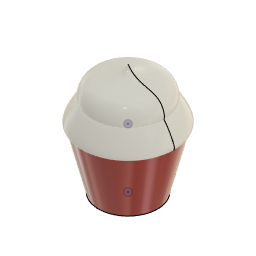
Cupcake v1 (Autodesk Fusion 360 design; units mm, degrees)
Autodesk Fusion 360 part; units mm, degrees
sketch "Sketch1" plane through (0, 0, 0) normal (0, 0, 1) x (1, 0, 0)
ref_plane "WorkPlane2" through (0, 0, 12.7) normal (0, 0, 1) x (1, 0, 0)
sketch "Sketch2" plane through (0, 0, 12.7) normal (0, 0, 1) x (1, 0, 0)
sketch "Sketch3" plane through (0, 0, 0) normal (0, 0, 1) x (1, 0, 0)
sketch "Sketch4" plane through (0, 0, 0) normal (0, 0, 1) x (1, 0, 0)
  circle A0 centre (0, 0) radius 6.35
  dimension "d5" = 12.7
  constraint coincident A0.centre origin
  measures "d5" diameter of A0
sketch "Sketch5" plane through (0, 0, 12.7) normal (0, 0, 1) x (1, 0, 0)
  circle A0 centre (0, 0) radius 9.525
  dimension "d6" = 19.05
  constraint coincident A0.centre origin
  measures "d6" diameter of A0
loft "Loft1" add profiles "Sketch5", "Sketch4" section 1 section 2 makes body 1
sketch "Sketch6" plane through (0, 0, 0) normal (0, 1, 0) x (1, 0, 0)
  line L0 (0.0062, -12.6962) -> (-9.4561, -12.6962)
  spline S0 degree 5 poles (-9.4561, -12.6962) (-9.6086, -12.5647) (-9.9028, -12.3297) (-10.3124, -12.0611) (-10.7944, -11.8716) (-11.2866, -11.9136) (-11.6595, -12.2218) (-11.8972, -12.7635) (-11.9766, -13.4827) (-11.8743, -14.3123) (-11.5728, -15.1831) (-11.0666, -16.0345) (-10.3696, -16.8243) (-9.5097, -17.5256) (-8.5237, -18.1236) (-7.4524, -18.6121) (-6.3357, -18.991) (-5.2079, -19.2636) (-4.0929, -19.4331) (-3.0059, -19.5033) (-1.9554, -19.4772) (-1.1474, -19.3813) (-0.56, -19.2678) (-0.1766, -19.1738) (0.013, -19.1222) knots 0 0 0 0 0 0 0.05 0.1 0.15 0.2 0.25 0.3 0.35 0.4 0.45 0.5 0.55 0.6 0.65 0.7 0.75 0.8 0.85 0.9 0.95 1 1 1 1 1 1
  line L1 (0.013, -19.1222) -> (0.0062, -12.6962)
  point P0 (-11.5402, -12.1763)
  point P1 (-11.5053, -15.213)
  point P2 (-6.2697, -18.9826)
  constraint horizontal L0
sketch "Sketch7" plane through (0, 0, 0) normal (1, 0, 0) x (0, 1, 0)
  line L0 (0.0682, 12.7183) -> (9.4407, 12.7183)
  spline S0 degree 5 poles (9.4407, 12.7183) (9.4977, 12.7532) (9.6081, 12.8323) (9.7632, 12.9784) (9.9492, 13.2281) (10.1441, 13.6298) (10.2936, 14.1146) (10.3826, 14.6695) (10.3846, 15.2722) (10.2702, 15.8937) (10.0166, 16.5023) (9.6175, 17.0677) (9.0923, 17.5644) (8.4968, 17.9753) (7.9308, 18.296) (7.5016, 18.5338) (7.2852, 18.7087) (7.2954, 18.8519) (7.4324, 19.0085) (7.4979, 19.2302) (7.3026, 19.5585) (6.766, 20.0073) (5.9102, 20.5648) (4.8251, 21.2012) (3.6437, 21.8737) (2.5134, 22.533) (1.5694, 23.1288) (0.9061, 23.6156) (0.5522, 23.9588) (0.4368, 24.1412) (0.379, 24.1666) (0.1829, 24.0491) (-0.2634, 23.8032) (-0.9835, 23.442) (-1.9389, 22.9788) (-3.0449, 22.4278) (-4.1907, 21.8052) (-5.2571, 21.1297) (-6.1358, 20.4238) (-6.7477, 19.7144) (-7.0623, 19.0342) (-7.1137, 18.4214) (-6.9775, 17.9116) (-6.7508, 17.5291) (-6.5312, 17.2791) (-6.3949, 17.1378) (-6.3819, 17.0498) (-6.513, 16.9543) (-6.8023, 16.8074) (-7.2591, 16.5802) (-7.8884, 16.2555) (-8.5318, 15.9111) (-9.0934, 15.6039) (-9.5028, 15.3775) (-9.7163, 15.2588) knots 0 0 0 0 0 0 0.02 0.04 0.06 0.08 0.1 0.12 0.14 0.16 0.18 0.2 0.22 0.24 0.26 0.28 0.3 0.32 0.34 0.36 0.38 0.4 0.42 0.44 0.46 0.48 0.5 0.52 0.54 0.56 0.58 0.6 0.62 0.64 0.66 0.68 0.7 0.72 0.74 0.76 0.78 0.8 0.82 0.84 0.86 0.88 0.9 0.92 0.94 0.96 0.98 1 1 1 1 1 1
  line L1 (0.3085, 24.1164) -> (0.0682, 12.7183)
  point P0 (10.299, 14.2289)
  point P1 (9.0974, 17.5247)
  point P2 (7.3121, 18.795)
  point P3 (7.4151, 19.31)
  point P4 (0.6518, 23.8761)
  point P5 (0.3085, 24.1164)
  point P6 (-6.6265, 19.7906)
  point P7 (-6.5922, 17.3531)
  point P8 (-6.4205, 17.0441)
  constraint horizontal L0
  constraint coincident P5 L1.start
sketch "Sketch8" plane through (0, 0, 0) normal (0, 1, 0) x (1, 0, 0)
  line L0 (-0.0077, -12.6935) -> (9.5283, -12.6935)
  spline S0 degree 5 poles (9.5283, -12.6935) (9.6108, -12.6817) (9.7571, -12.6787) (9.9205, -12.7363) (10.0259, -12.9376) (9.9748, -13.3889) (9.7568, -14.015) (9.4058, -14.7629) (8.9773, -15.5472) (8.5361, -16.2724) (8.1459, -16.8519) (7.8587, -17.228) (7.7042, -17.3916) (7.6789, -17.4018) (7.7344, -17.4088) (7.8043, -17.564) (7.8346, -17.9155) (7.7851, -18.4332) (7.6282, -19.0425) (7.3494, -19.6531) (6.947, -20.1927) (6.4316, -20.6291) (5.8224, -20.9582) (5.1448, -21.1974) (4.4268, -21.3784) (3.6968, -21.5396) (2.9802, -21.7189) (2.2965, -21.9457) (1.6587, -22.2399) (1.0755, -22.6147) (0.5517, -23.0771) (0.1818, -23.5198) (-0.0677, -23.8931) (-0.2216, -24.1602) (-0.2955, -24.2984) knots 0 0 0 0 0 0 0.033333 0.066667 0.1 0.133333 0.166667 0.2 0.233333 0.266667 0.3 0.333333 0.366667 0.4 0.433333 0.466667 0.5 0.533333 0.566667 0.6 0.633333 0.666667 0.7 0.733333 0.766667 0.8 0.833333 0.866667 0.9 0.933333 0.966667 1 1 1 1 1 1
  line L1 (-0.0077, -12.6935) -> (-0.0077, -23.816)
  point P0 (9.7817, -13.8999)
  point P1 (7.7319, -17.3584)
  point P2 (7.7427, -17.4525)
  point P3 (7.4038, -19.4837)
  point P4 (3.4796, -21.598)
  constraint horizontal L0
  constraint coincident S0 L1.end
  constraint perpendicular L0 L1
revolve "Revolve3" add sketch "Sketch8" angle 360 about axis through (-0.0077, 0, 12.6935) along (0, 0, 1) separate body makes body 2
